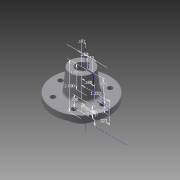
# Autodesk Inventor part: denso-6 coupler
Saved by Autodesk Inventor 2015 (Build 190159000, 159)
## iProperties
Created: 2015-02-04
Part Number: denso-6 coupler
Material: Generic
Document SubType Name: Modeling
Designer: sethbattis
Density: 1 g/cm^3
Appearance: Default
Author: sethbattis
Autodesk Inventor part; units mm, degrees
ref_plane "YZ Plane" through (0, 0, 0) normal (1, 0, 0) x (0, 1, 0)
ref_plane "XZ Plane" through (0, 0, 0) normal (0, 1, 0) x (-1, 0, 0)
ref_plane "XY Plane" through (0, 0, 0) normal (0, 0, 1) x (1, 0, 0)
sketch "Sketch1" plane through (0, 0, 0) normal (0, 0, 1) x (1, 0, 0)
  line L0 (0, 0) -> (0, 50.8) construction
  line L1 (0, 0) -> (50.8, 0) construction
  line L2 (0, 50.8) -> (6.35, 50.8) construction
  line L3 (6.35, 50.8) -> (6.35, 0) construction
  line L4 (6.35, 50.8) -> (12.7, 50.8)
  line L5 (0, 25.6759) -> (14.9225, 25.6759) construction
  line L6 (12.7, 50.8) -> (14.9225, 25.6759)
  line L7 (0, 19.2751) -> (31.75, 19.2751) construction
  line L8 (31.75, 19.2751) -> (31.75, 25.6759)
  line L9 (14.9225, 25.6759) -> (31.75, 25.6759)
  line L10 (0, 9.5479) -> (15.8115, 9.5479) construction
  line L11 (31.75, 19.2751) -> (15.875, 19.2751)
  line L12 (15.875, 19.2751) -> (15.875, 6.5751)
  line L13 (15.875, 19.2751) -> (28.575, 19.2751) construction
  line L14 (0, 22.4755) -> (31.75, 22.4755) construction
  line L15 (6.35, 50.8) -> (6.35, 25.6759)
  line L16 (0, 6.5751) -> (8.2867, 6.5751) construction
  line L17 (8.2867, 6.5751) -> (15.875, 6.5751)
  line L18 (8.2867, 6.5751) -> (8.2867, 19.2751)
  line L19 (23.5585, 11.9908) -> (23.5585, 41.3472) construction
  line L20 (4.5974, 71.0633) -> (4.5974, -11.3243) construction
  line L21 (8.2867, 19.2751) -> (4.5974, 19.2751)
  line L22 (4.5974, 25.6759) -> (6.35, 25.6759)
  line L23 (4.5974, 25.6759) -> (4.5974, 19.2751)
  dimension "d2" = 50.8
  dimension "d3" = 90
  dimension "d4" = 6.35
  dimension "d5" = 6.35
  dimension "d6" = 14.9225
  dimension "d8" = 25.2222
  dimension "d9" = 31.75
  dimension "d11" = 6.4008
  dimension "d12" = 15.8115
  dimension "d13" = 12.7
  dimension "d14" = 90
  dimension "d15" = 8.2867
  dimension "d28" = 8.1915
  dimension "d55" = 4.5974
  dimension "d56" = 12.7
  dimension "d57" = 25.1241
  constraints: 50 end point, 12 point on line, 7 horizontal, 7 perpendicular, 4 vertical, 2 midpoint, 1 collinear, 1 horizontal alignment, 1 parallel
  measures "d2" distance of L0.start L0.end
  measures "d3" angle of L1 L0
  measures "d4" distance of L0.end L2.end
  measures "d5" distance of L2.end L4.end
  measures "d6" distance of L5.start L5.end
  measures "d8" distance of L4.end L5.end
  measures "d9" distance of L7.start L7.end
  measures "d11" distance of L7.end L8.end
  measures "d12" distance of L10.start L10.end
  measures "d13" distance of L11.end L12.end
  measures "d14" angle of L12 L13
  measures "d15" distance of L16.start L16.end
  measures "d28" distance between parallel lines of L8 L19
  measures "d55" distance between parallel lines of L0 L20
  measures "d56" distance of L16.end L18.end
  measures "d57" distance of L2.end L15.end
revolve "Revolution1" add sketch "Sketch1" angle 360 about axis through (0, 0, 0) along (0, 1, 0)
fillet "Fillet1" radius 3.175 1 edges at (-14.9225, 25.6759, 0)
fillet "Fillet2" radius 3.175 1 edges at (-15.875, 19.2751, 0)
hole "Hole2" at (23.4944, 25.6759, -0.034) direction (0, -1, 0) diameter 5.3975 end through all
pattern_circular "Circular Pattern1" count 6 over 360 about axis through (0, 38.238, 0) along (0, -1, 0) of "Hole2"
sketch "Sketch2" plane through (0, 6.5751, 0) normal (0, -1, 0) x (1, 0, 0)
  circle A0 centre (0, 0) radius 8.2867 construction
  line L0 (-2.2055, 7.9879) -> (-2.2121, 9.8928)
  circle A1 centre (0, 0) radius 10.1371 construction
  line L1 (2.1506, 8.0028) -> (2.144, 9.9078)
  line L2 (-2.2055, 7.9879) -> (2.1506, 8.0028) construction
  arc A2 (2.144, 9.9078) -> (-2.2121, 9.8928) centre (0, 0) ccw
  arc A3 (2.1506, 8.0028) -> (-2.2055, 7.9879) centre (0, 0) ccw
  dimension "d43" = 1.905
  dimension "d44" = 4.3561
  constraints: 8 point on circle, 6 end point, 3 centre point, 2 coincident, 2 perpendicular, 1 concentric
  measures "d43" distance of L0.start L0.end
  measures "d44" distance of L0.start L1.start
extrude "Extrusion1" cut sketch "Sketch2" against normal blind 12.7
pattern_circular "Circular Pattern2" count 6 over 360 about axis through (0, 12.9251, 0) along (0, -1, 0) of "Extrusion1"
sketch "Sketch3" plane through (0, 50.8, 0) normal (0, 1, 0) x (1, 0, 0)
  circle A0 centre (0, 0) radius 6.35 construction
  line L0 (0, 6.35) -> (0, 8.128) construction
  circle A1 centre (0, 0) radius 8.128 construction
  line L1 (-1.5685, 6.1532) -> (-2.0076, 7.8762)
  line L2 (1.5685, 6.1532) -> (2.0076, 7.8762)
  line L3 (-1.5685, 6.1532) -> (1.5685, 6.1532) construction
  arc A2 (2.0076, 7.8762) -> (-2.0076, 7.8762) centre (0, 0) ccw
  arc A3 (1.5685, 6.1532) -> (-1.5685, 6.1532) centre (0, 0) ccw
  dimension "d51" = 1.778
  dimension "d52" = 3.1369
  constraints: 10 point on circle, 8 end point, 3 centre point, 3 line through centre, 2 concentric, 1 coincident, 1 vertical, 1 other
  measures "d51" distance of L0.start L0.end
  measures "d52" distance of L1.start L2.start
extrude "Extrusion2" cut sketch "Sketch3" against normal blind 25.1206
body "Solid1"
